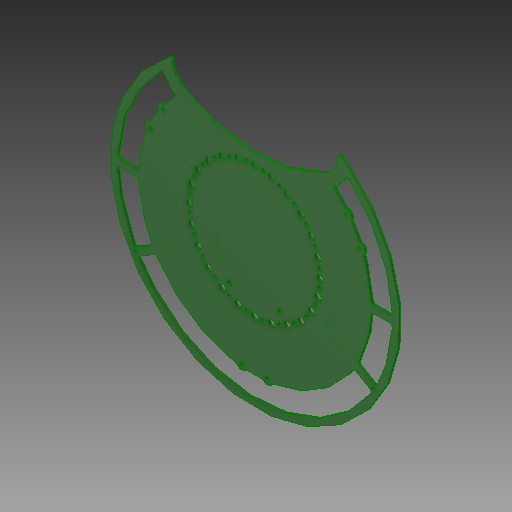
# Autodesk Inventor part: Board 0.brd_Outline
Saved by Autodesk Inventor 2017 (Build 210142000, 142)
## iProperties
Created: 2019-06-13
Part Number: Board 0.brd_Outline
Material: Generic
Document SubType Name: Modeling
Designer: Marc
Density: 1 g/cm^3
Appearance: Board Outline
Author: Marc
Autodesk Inventor part; units mm, degrees
ref_plane "YZ Plane" through (0, 0, 0) normal (1, 0, 0) x (0, 1, 0)
ref_plane "XZ Plane" through (0, 0, 0) normal (0, 1, 0) x (-1, 0, 0)
ref_plane "XY Plane" through (0, 0, 0) normal (0, 0, 1) x (1, 0, 0)
sketch "Sketch1" plane through (0, 0, 0) normal (0, 0, 1) x (1, 0, 0)
  line L0 (-60.7484, 83.79) -> (-60.8086, 84.044)
  line L1 (-60.8086, 84.044) -> (-60.9324, 84.2738)
  line L2 (-60.9324, 84.2738) -> (-61.1115, 84.4637)
  line L3 (-61.1115, 84.4637) -> (-61.3337, 84.6008)
  line L4 (-61.3337, 84.6008) -> (-61.5837, 84.6757)
  line L5 (-61.5837, 84.6757) -> (-61.8447, 84.6834)
  line L6 (-61.8447, 84.6834) -> (-62.0987, 84.6232)
  line L7 (-62.0987, 84.6232) -> (-62.3285, 84.4994)
  line L8 (-62.3285, 84.4994) -> (-62.337, 84.4932)
  line L9 (-62.337, 84.4932) -> (-82.0805, 65.4803)
  line L10 (-82.0805, 65.4803) -> (-96.2304, 42.0052)
  line L11 (-96.2304, 42.0052) -> (-103.8223, 15.6678)
  line L12 (-103.8223, 15.6678) -> (-104.339, -11.7372)
  line L13 (-104.339, -11.7372) -> (-97.7451, -38.342)
  line L14 (-97.7451, -38.342) -> (-84.49, -62.3337)
  line L15 (-84.49, -62.3337) -> (-65.4771, -82.0773)
  line L16 (-65.4771, -82.0773) -> (-42.002, -96.2272)
  line L17 (-42.002, -96.2272) -> (-15.6646, -103.8191)
  line L18 (-15.6646, -103.8191) -> (11.7404, -104.3358)
  line L19 (11.7404, -104.3358) -> (38.3452, -97.7419)
  line L20 (38.3452, -97.7419) -> (62.3369, -84.4868)
  line L21 (62.3369, -84.4868) -> (82.0805, -65.4739)
  line L22 (82.0805, -65.4739) -> (96.2304, -41.9988)
  line L23 (96.2304, -41.9988) -> (103.8223, -15.6614)
  line L24 (103.8223, -15.6614) -> (104.339, 11.7436)
  line L25 (104.339, 11.7436) -> (97.7451, 38.3484)
  line L26 (97.7451, 38.3484) -> (84.49, 62.3401)
  line L27 (84.49, 62.3401) -> (65.4771, 82.0837)
  line L28 (65.4771, 82.0837) -> (62.337, 84.4932)
  line L29 (62.337, 84.4932) -> (62.1085, 84.6195)
  line L30 (62.1085, 84.6195) -> (61.8551, 84.6823)
  line L31 (61.8551, 84.6823) -> (61.5941, 84.6773)
  line L32 (61.5941, 84.6773) -> (61.3432, 84.605)
  line L33 (61.3432, 84.605) -> (61.1197, 84.4703)
  line L34 (61.1197, 84.4703) -> (60.9386, 84.2823)
  line L35 (60.9386, 84.2823) -> (60.8123, 84.0538)
  line L36 (60.8123, 84.0538) -> (60.7495, 83.8004)
  line L37 (60.7495, 83.8004) -> (60.7484, 83.79)
  line L38 (60.7484, 83.79) -> (59.5017, 78.5255)
  line L39 (59.5017, 78.5255) -> (56.935, 73.7631)
  line L40 (56.935, 73.7631) -> (53.2231, 69.8273)
  line L41 (53.2231, 69.8273) -> (50, 67.6691)
  line L42 (50, 67.6691) -> (24.3974, 57.8745)
  line L43 (24.3974, 57.8745) -> (-2.8678, 55.04)
  line L44 (-2.8678, 55.04) -> (-29.9376, 59.359)
  line L45 (-29.9376, 59.359) -> (-50, 67.6691)
  line L46 (-50, 67.6691) -> (-54.3803, 70.8442)
  line L47 (-54.3803, 70.8442) -> (-57.7896, 75.0449)
  line L48 (-57.7896, 75.0449) -> (-59.9955, 79.9848)
  line L49 (-59.9955, 79.9848) -> (-60.7484, 83.79)
  line L50 (-83.531, -51.1134) -> (-73.5598, -45.3565)
  line L51 (-73.5598, -45.3565) -> (-73.0774, -45.1567)
  line L52 (-73.0774, -45.1567) -> (-72.5598, -45.0885)
  line L53 (-72.5598, -45.0885) -> (-72.0422, -45.1567)
  line L54 (-72.0422, -45.1567) -> (-71.5598, -45.3565)
  line L55 (-71.5598, -45.3565) -> (-71.1456, -45.6743)
  line L56 (-71.1456, -45.6743) -> (-70.8821, -45.9998)
  line L57 (-70.8821, -45.9998) -> (-56.5631, -62.7771)
  line L58 (-56.5631, -62.7771) -> (-38.3898, -75.2767)
  line L59 (-38.3898, -75.2767) -> (-17.6006, -82.6468)
  line L60 (-17.6006, -82.6468) -> (-13.0912, -83.4798)
  line L61 (-13.0912, -83.4798) -> (-12.5816, -84.3912)
  line L62 (-12.5816, -84.3912) -> (-11.8534, -85.1396)
  line L63 (-11.8534, -85.1396) -> (-10.9564, -85.6741)
  line L64 (-10.9564, -85.6741) -> (-9.9515, -85.9582)
  line L65 (-9.9515, -85.9582) -> (-8.9074, -85.9725)
  line L66 (-8.9074, -85.9725) -> (-7.8952, -85.7162)
  line L67 (-7.8952, -85.7162) -> (-6.9838, -85.2065)
  line L68 (-6.9838, -85.2065) -> (-6.2353, -84.4784)
  line L69 (-6.2353, -84.4784) -> (-6.0887, -84.2803)
  line L70 (-6.0887, -84.2803) -> (6.0887, -84.2803)
  line L71 (6.0887, -84.2803) -> (6.7909, -85.0532)
  line L72 (6.7909, -85.0532) -> (7.6692, -85.618)
  line L73 (7.6692, -85.618) -> (8.6637, -85.9362)
  line L74 (8.6637, -85.9362) -> (9.7067, -85.9862)
  line L75 (9.7067, -85.9862) -> (10.7271, -85.7645)
  line L76 (10.7271, -85.7645) -> (11.6554, -85.2863)
  line L77 (11.6554, -85.2863) -> (12.4283, -84.5841)
  line L78 (12.4283, -84.5841) -> (12.9931, -83.7058)
  line L79 (12.9931, -83.7058) -> (13.0912, -83.4798)
  line L80 (13.0912, -83.4798) -> (34.2497, -77.2484)
  line L81 (34.2497, -77.2484) -> (53.0744, -65.7531)
  line L82 (53.0744, -65.7531) -> (68.2824, -49.7774)
  line L83 (68.2824, -49.7774) -> (70.8821, -45.9998)
  line L84 (70.8821, -45.9998) -> (71.221, -45.6027)
  line L85 (71.221, -45.6027) -> (71.6512, -45.3068)
  line L86 (71.6512, -45.3068) -> (72.1433, -45.1324)
  line L87 (72.1433, -45.1324) -> (72.6638, -45.0912)
  line L88 (72.6638, -45.0912) -> (73.1771, -45.1862)
  line L89 (73.1771, -45.1862) -> (73.5598, -45.3565)
  line L90 (73.5598, -45.3565) -> (83.531, -51.1134)
  line L91 (83.531, -51.1134) -> (83.9452, -51.4312)
  line L92 (83.9452, -51.4312) -> (84.263, -51.8455)
  line L93 (84.263, -51.8455) -> (84.4628, -52.3278)
  line L94 (84.4628, -52.3278) -> (84.531, -52.8455)
  line L95 (84.531, -52.8455) -> (84.4628, -53.3631)
  line L96 (84.4628, -53.3631) -> (84.263, -53.8455)
  line L97 (84.263, -53.8455) -> (84.2153, -53.9239)
  line L98 (84.2153, -53.9239) -> (67.3902, -73.8831)
  line L99 (67.3902, -73.8831) -> (45.9725, -88.8076)
  line L100 (45.9725, -88.8076) -> (21.4219, -97.6803)
  line L101 (21.4219, -97.6803) -> (-4.5885, -99.8964)
  line L102 (-4.5885, -99.8964) -> (-30.2863, -95.3051)
  line L103 (-30.2863, -95.3051) -> (-53.9201, -84.2191)
  line L104 (-53.9201, -84.2191) -> (-73.8793, -67.394)
  line L105 (-73.8793, -67.394) -> (-84.2153, -53.9239)
  line L106 (-84.2153, -53.9239) -> (-84.437, -53.4512)
  line L107 (-84.437, -53.4512) -> (-84.5288, -52.9373)
  line L108 (-84.5288, -52.9373) -> (-84.4845, -52.417)
  line L109 (-84.4845, -52.417) -> (-84.3071, -51.926)
  line L110 (-84.3071, -51.926) -> (-84.0086, -51.4976)
  line L111 (-84.0086, -51.4976) -> (-83.6094, -51.1611)
  line L112 (-83.6094, -51.1611) -> (-83.531, -51.1134)
  line L113 (-76.0333, 36.8672) -> (-77.0537, 36.6456)
  line L114 (-77.0537, 36.6456) -> (-77.9819, 36.1673)
  line L115 (-77.9819, 36.1673) -> (-78.7548, 35.4651)
  line L116 (-78.7548, 35.4651) -> (-79.3196, 34.5868)
  line L117 (-79.3196, 34.5868) -> (-79.6378, 33.5923)
  line L118 (-79.6378, 33.5923) -> (-79.6878, 32.5492)
  line L119 (-79.6878, 32.5492) -> (-79.4661, 31.5288)
  line L120 (-79.4661, 31.5288) -> (-78.9878, 30.6006)
  line L121 (-78.9878, 30.6006) -> (-78.8412, 30.4026)
  line L122 (-78.8412, 30.4026) -> (-84.0231, 8.9665)
  line L123 (-84.0231, 8.9665) -> (-84.3856, 4.396)
  line L124 (-84.3856, 4.396) -> (-84.4806, 3.8826)
  line L125 (-84.4806, 3.8826) -> (-84.7052, 3.4113)
  line L126 (-84.7052, 3.4113) -> (-85.0441, 3.0141)
  line L127 (-85.0441, 3.0141) -> (-85.4743, 2.7183)
  line L128 (-85.4743, 2.7183) -> (-85.9664, 2.5438)
  line L129 (-85.9664, 2.5438) -> (-86.3829, 2.5)
  line L130 (-86.3829, 2.5) -> (-97.8966, 2.5)
  line L131 (-97.8966, 2.5) -> (-98.4143, 2.5682)
  line L132 (-98.4143, 2.5682) -> (-98.8966, 2.768)
  line L133 (-98.8966, 2.768) -> (-99.3109, 3.0858)
  line L134 (-99.3109, 3.0858) -> (-99.6287, 3.5)
  line L135 (-99.6287, 3.5) -> (-99.8285, 3.9824)
  line L136 (-99.8285, 3.9824) -> (-99.8966, 4.5001)
  line L137 (-99.8966, 4.5001) -> (-99.8945, 4.5918)
  line L138 (-99.8945, 4.5918) -> (-95.3026, 30.2894)
  line L139 (-95.3026, 30.2894) -> (-84.2162, 53.9228)
  line L140 (-84.2162, 53.9228) -> (-68.6444, 72.7182)
  line L141 (-68.6444, 72.7182) -> (-68.2212, 73.024)
  line L142 (-68.2212, 73.024) -> (-67.7333, 73.2098)
  line L143 (-67.7333, 73.2098) -> (-67.2139, 73.263)
  line L144 (-67.2139, 73.263) -> (-66.6984, 73.1799)
  line L145 (-66.6984, 73.1799) -> (-66.222, 72.9663)
  line L146 (-66.222, 72.9663) -> (-65.8171, 72.6366)
  line L147 (-65.8171, 72.6366) -> (-65.5113, 72.2134)
  line L148 (-65.5113, 72.2134) -> (-65.511, 72.2128)
  line L149 (-65.511, 72.2128) -> (-61.1063, 66.1109)
  line L150 (-61.1063, 66.1109) -> (-59.4525, 64.4927)
  line L151 (-59.4525, 64.4927) -> (-58.8449, 64.1171)
  line L152 (-58.8449, 64.1171) -> (-58.4393, 63.7882)
  line L153 (-58.4393, 63.7882) -> (-58.1327, 63.3656)
  line L154 (-58.1327, 63.3656) -> (-57.9459, 62.8781)
  line L155 (-57.9459, 62.8781) -> (-57.8917, 62.3588)
  line L156 (-57.8917, 62.3588) -> (-57.9738, 61.8431)
  line L157 (-57.9738, 61.8431) -> (-58.1865, 61.3663)
  line L158 (-58.1865, 61.3663) -> (-58.5062, 60.9694)
  line L159 (-58.5062, 60.9694) -> (-65.75, 53.0772)
  line L160 (-65.75, 53.0772) -> (-66.7941, 53.0916)
  line L161 (-66.7941, 53.0916) -> (-67.8064, 52.8352)
  line L162 (-67.8064, 52.8352) -> (-68.7178, 52.3255)
  line L163 (-68.7178, 52.3255) -> (-69.4662, 51.5974)
  line L164 (-69.4662, 51.5974) -> (-70.0007, 50.7003)
  line L165 (-70.0007, 50.7003) -> (-70.2848, 49.6955)
  line L166 (-70.2848, 49.6955) -> (-70.2991, 48.6514)
  line L167 (-70.2991, 48.6514) -> (-70.0428, 47.6391)
  line L168 (-70.0428, 47.6391) -> (-69.9446, 47.4131)
  line L169 (-69.9446, 47.4131) -> (-76.0333, 36.8672)
  line L170 (97.8966, 2.5) -> (86.3829, 2.5)
  line L171 (86.3829, 2.5) -> (85.8652, 2.5681)
  line L172 (85.8652, 2.5681) -> (85.3829, 2.7679)
  line L173 (85.3829, 2.7679) -> (84.9687, 3.0857)
  line L174 (84.9687, 3.0857) -> (84.6508, 3.4999)
  line L175 (84.6508, 3.4999) -> (84.451, 3.9823)
  line L176 (84.451, 3.9823) -> (84.3856, 4.396)
  line L177 (84.3856, 4.396) -> (80.3743, 26.0815)
  line L178 (80.3743, 26.0815) -> (78.8412, 30.4026)
  line L179 (78.8412, 30.4026) -> (79.3757, 31.2996)
  line L180 (79.3757, 31.2996) -> (79.6598, 32.3044)
  line L181 (79.6598, 32.3044) -> (79.6741, 33.3486)
  line L182 (79.6741, 33.3486) -> (79.4177, 34.3608)
  line L183 (79.4177, 34.3608) -> (78.9081, 35.2722)
  line L184 (78.9081, 35.2722) -> (78.18, 36.0207)
  line L185 (78.18, 36.0207) -> (77.2829, 36.5552)
  line L186 (77.2829, 36.5552) -> (76.2781, 36.8393)
  line L187 (76.2781, 36.8393) -> (76.0333, 36.8672)
  line L188 (76.0333, 36.8672) -> (69.9446, 47.4131)
  line L189 (69.9446, 47.4131) -> (70.2628, 48.4077)
  line L190 (70.2628, 48.4077) -> (70.3128, 49.4507)
  line L191 (70.3128, 49.4507) -> (70.0911, 50.4711)
  line L192 (70.0911, 50.4711) -> (69.6129, 51.3994)
  line L193 (69.6129, 51.3994) -> (68.9107, 52.1722)
  line L194 (68.9107, 52.1722) -> (68.0324, 52.737)
  line L195 (68.0324, 52.737) -> (67.0378, 53.0552)
  line L196 (67.0378, 53.0552) -> (65.9948, 53.1052)
  line L197 (65.9948, 53.1052) -> (65.75, 53.0772)
  line L198 (65.75, 53.0772) -> (58.5062, 60.9694)
  line L199 (58.5062, 60.9694) -> (58.1799, 61.377)
  line L200 (58.1799, 61.377) -> (57.9702, 61.8552)
  line L201 (57.9702, 61.8552) -> (57.8914, 62.3713)
  line L202 (57.8914, 62.3713) -> (57.9489, 62.8903)
  line L203 (57.9489, 62.8903) -> (58.1387, 63.3766)
  line L204 (58.1387, 63.3766) -> (58.448, 63.7973)
  line L205 (58.448, 63.7973) -> (58.8449, 64.1171)
  line L206 (58.8449, 64.1171) -> (59.4525, 64.4927)
  line L207 (59.4525, 64.4927) -> (64.3323, 70.2217)
  line L208 (64.3323, 70.2217) -> (65.511, 72.2128)
  line L209 (65.511, 72.2128) -> (65.8166, 72.6361)
  line L210 (65.8166, 72.6361) -> (66.2214, 72.9659)
  line L211 (66.2214, 72.9659) -> (66.6977, 73.1797)
  line L212 (66.6977, 73.1797) -> (67.2132, 73.263)
  line L213 (67.2132, 73.263) -> (67.7326, 73.21)
  line L214 (67.7326, 73.21) -> (68.2206, 73.0243)
  line L215 (68.2206, 73.0243) -> (68.6439, 72.7187)
  line L216 (68.6439, 72.7187) -> (68.6444, 72.7182)
  line L217 (68.6444, 72.7182) -> (85.1261, 52.4746)
  line L218 (85.1261, 52.4746) -> (95.8067, 28.655)
  line L219 (95.8067, 28.655) -> (99.8945, 4.5918)
  line L220 (99.8945, 4.5918) -> (99.8502, 4.0716)
  line L221 (99.8502, 4.0716) -> (99.6728, 3.5806)
  line L222 (99.6728, 3.5806) -> (99.3743, 3.1522)
  line L223 (99.3743, 3.1522) -> (98.9751, 2.8157)
  line L224 (98.9751, 2.8157) -> (98.5024, 2.5939)
  line L225 (98.5024, 2.5939) -> (97.9884, 2.5021)
  line L226 (97.9884, 2.5021) -> (97.8966, 2.5)
  line L227 (-97.8966, -2.5) -> (-86.3829, -2.5)
  line L228 (-86.3829, -2.5) -> (-85.8652, -2.5681)
  line L229 (-85.8652, -2.5681) -> (-85.3829, -2.7679)
  line L230 (-85.3829, -2.7679) -> (-84.9687, -3.0857)
  line L231 (-84.9687, -3.0857) -> (-84.6508, -3.4999)
  line L232 (-84.6508, -3.4999) -> (-84.451, -3.9823)
  line L233 (-84.451, -3.9823) -> (-84.3856, -4.396)
  line L234 (-84.3856, -4.396) -> (-80.3739, -26.0833)
  line L235 (-80.3739, -26.0833) -> (-75.278, -38.3858)
  line L236 (-75.278, -38.3858) -> (-75.1036, -38.8779)
  line L237 (-75.1036, -38.8779) -> (-75.0625, -39.3983)
  line L238 (-75.0625, -39.3983) -> (-75.1574, -39.9117)
  line L239 (-75.1574, -39.9117) -> (-75.382, -40.383)
  line L240 (-75.382, -40.383) -> (-75.721, -40.7802)
  line L241 (-75.721, -40.7802) -> (-76.0598, -41.0264)
  line L242 (-76.0598, -41.0264) -> (-86.031, -46.7833)
  line L243 (-86.031, -46.7833) -> (-86.5133, -46.983)
  line L244 (-86.5133, -46.983) -> (-87.031, -47.0512)
  line L245 (-87.031, -47.0512) -> (-87.5486, -46.983)
  line L246 (-87.5486, -46.983) -> (-88.031, -46.7832)
  line L247 (-88.031, -46.7832) -> (-88.4452, -46.4654)
  line L248 (-88.4452, -46.4654) -> (-88.763, -46.0511)
  line L249 (-88.763, -46.0511) -> (-88.8071, -45.9706)
  line L250 (-88.8071, -45.9706) -> (-97.6786, -21.4231)
  line L251 (-97.6786, -21.4231) -> (-99.8945, -4.5918)
  line L252 (-99.8945, -4.5918) -> (-99.8502, -4.0716)
  line L253 (-99.8502, -4.0716) -> (-99.6728, -3.5806)
  line L254 (-99.6728, -3.5806) -> (-99.3743, -3.1522)
  line L255 (-99.3743, -3.1522) -> (-98.9751, -2.8157)
  line L256 (-98.9751, -2.8157) -> (-98.5024, -2.5939)
  line L257 (-98.5024, -2.5939) -> (-97.9884, -2.5021)
  line L258 (-97.9884, -2.5021) -> (-97.8966, -2.5)
  line L259 (86.031, -46.7833) -> (76.0598, -41.0264)
  line L260 (76.0598, -41.0264) -> (75.6456, -40.7085)
  line L261 (75.6456, -40.7085) -> (75.3277, -40.2943)
  line L262 (75.3277, -40.2943) -> (75.1279, -39.812)
  line L263 (75.1279, -39.812) -> (75.0597, -39.2944)
  line L264 (75.0597, -39.2944) -> (75.1279, -38.7767)
  line L265 (75.1279, -38.7767) -> (75.278, -38.3858)
  line L266 (75.278, -38.3858) -> (82.6475, -17.5982)
  line L267 (82.6475, -17.5982) -> (84.3856, -4.396)
  line L268 (84.3856, -4.396) -> (84.4806, -3.8826)
  line L269 (84.4806, -3.8826) -> (84.7052, -3.4113)
  line L270 (84.7052, -3.4113) -> (85.0441, -3.0141)
  line L271 (85.0441, -3.0141) -> (85.4743, -2.7183)
  line L272 (85.4743, -2.7183) -> (85.9664, -2.5438)
  line L273 (85.9664, -2.5438) -> (86.3829, -2.5)
  line L274 (86.3829, -2.5) -> (97.8966, -2.5)
  line L275 (97.8966, -2.5) -> (98.4143, -2.5682)
  line L276 (98.4143, -2.5682) -> (98.8966, -2.768)
  line L277 (98.8966, -2.768) -> (99.3109, -3.0858)
  line L278 (99.3109, -3.0858) -> (99.6287, -3.5)
  line L279 (99.6287, -3.5) -> (99.8285, -3.9824)
  line L280 (99.8285, -3.9824) -> (99.8966, -4.5001)
  line L281 (99.8966, -4.5001) -> (99.8945, -4.5918)
  line L282 (99.8945, -4.5918) -> (95.3037, -30.2863)
  line L283 (95.3037, -30.2863) -> (88.8071, -45.9706)
  line L284 (88.8071, -45.9706) -> (88.5086, -46.399)
  line L285 (88.5086, -46.399) -> (88.1094, -46.7355)
  line L286 (88.1094, -46.7355) -> (87.6367, -46.9572)
  line L287 (87.6367, -46.9572) -> (87.1228, -47.0491)
  line L288 (87.1228, -47.0491) -> (86.6025, -47.0048)
  line L289 (86.6025, -47.0048) -> (86.1115, -46.8273)
  line L290 (86.1115, -46.8273) -> (86.031, -46.7833)
  circle A0 centre (-75.7016, 32.881) radius 1.5
  circle A1 centre (-66.3266, 49.119) radius 1.5
  circle A2 centre (66.3266, 49.119) radius 1.5
  circle A3 centre (75.7016, 32.881) radius 1.5
  circle A4 centre (86.5112, -49.9473) radius 1.5
  circle A5 centre (-86.5112, -49.9473) radius 1.5
  circle A6 centre (-9.375, -82) radius 1.5
  circle A7 centre (9.375, -82) radius 1.5
  circle A8 centre (-18.1775, -35.3843) radius 1.5
  circle A9 centre (18.1775, -35.3843) radius 1.5
  circle A10 centre (-47.0936, 6.2) radius 1.55
  circle A11 centre (-43.8843, 18.1775) radius 1.55
  circle A12 centre (-37.6843, 28.9162) radius 1.55
  circle A13 centre (-28.9162, 37.6843) radius 1.55
  circle A14 centre (-18.1775, 43.8843) radius 1.55
  circle A15 centre (-6.2, 47.0936) radius 1.55
  circle A16 centre (-6.2, -47.0936) radius 1.55
  circle A17 centre (-18.1775, -43.8843) radius 1.55
  circle A18 centre (-28.9162, -37.6843) radius 1.55
  circle A19 centre (-37.6843, -28.9162) radius 1.55
  circle A20 centre (-43.8843, -18.1775) radius 1.55
  circle A21 centre (-47.0936, -6.2) radius 1.55
  circle A22 centre (47.0936, -6.2) radius 1.55
  circle A23 centre (43.8843, -18.1775) radius 1.55
  circle A24 centre (37.6843, -28.9162) radius 1.55
  circle A25 centre (28.9162, -37.6843) radius 1.55
  circle A26 centre (18.1775, -43.8843) radius 1.55
  circle A27 centre (6.2, -47.0936) radius 1.55
  circle A28 centre (6.2, 47.0936) radius 1.55
  circle A29 centre (18.1775, 43.8843) radius 1.55
  circle A30 centre (28.9162, 37.6843) radius 1.55
  circle A31 centre (37.6843, 28.9162) radius 1.55
  circle A32 centre (43.8843, 18.1775) radius 1.55
  circle A33 centre (47.0936, 6.2) radius 1.55
  circle A34 centre (-47.5, 0) radius 2.5
  circle A35 centre (-45.8815, 12.2939) radius 2.5
  circle A36 centre (-41.1362, 23.75) radius 2.5
  circle A37 centre (-33.5876, 33.5876) radius 2.5
  circle A38 centre (-23.75, 41.1362) radius 2.5
  circle A39 centre (-12.2939, 45.8815) radius 2.5
  circle A40 centre (0, -47.5) radius 2.5
  circle A41 centre (-12.2939, -45.8815) radius 2.5
  circle A42 centre (-23.75, -41.1362) radius 2.5
  circle A43 centre (-33.5876, -33.5876) radius 2.5
  circle A44 centre (-41.1362, -23.75) radius 2.5
  circle A45 centre (-45.8815, -12.2939) radius 2.5
  circle A46 centre (47.5, 0) radius 2.5
  circle A47 centre (45.8815, -12.2939) radius 2.5
  circle A48 centre (41.1362, -23.75) radius 2.5
  circle A49 centre (33.5876, -33.5876) radius 2.5
  circle A50 centre (23.75, -41.1362) radius 2.5
  circle A51 centre (12.2939, -45.8815) radius 2.5
  circle A52 centre (0, 47.5) radius 2.5
  circle A53 centre (12.2939, 45.8815) radius 2.5
  circle A54 centre (23.75, 41.1362) radius 2.5
  circle A55 centre (33.5876, 33.5876) radius 2.5
  circle A56 centre (41.1362, 23.75) radius 2.5
  circle A57 centre (45.8815, 12.2939) radius 2.5
  circle A58 centre (-38.1762, -33.7185) radius 0.3048
  circle A59 centre (-36.6903, -42.4053) radius 0.3048
  circle A60 centre (-24.2316, -48.4632) radius 0.3048
  circle A61 centre (-31.4325, -51.2064) radius 0.3048
  circle A62 centre (-72.1233, -21.9456) radius 0.3048
  circle A63 centre (-73.9521, -20.1168) radius 0.3048
  circle A64 centre (-56.4642, -5.715) radius 0.3048
  circle A65 centre (-60.2361, -5.715) radius 0.3048
  circle A66 centre (-54.6354, 6.6294) radius 0.3048
  circle A67 centre (-51.435, -17.145) radius 0.3048
  circle A68 centre (-57.9501, 13.8303) radius 0.3048
  circle A69 centre (52.2351, -27.8892) radius 0.3048
  circle A70 centre (52.2351, -25.8318) radius 0.3048
  circle A71 centre (48.9204, -33.6042) radius 0.3048
  circle A72 centre (-23.2029, -24.2316) radius 0.3048
  circle A73 centre (-26.5176, -19.431) radius 0.3048
  circle A74 centre (58.5216, -33.6042) radius 0.175
  circle A75 centre (1.2573, -56.2356) radius 0.175
  circle A76 centre (57.15, -32.1183) radius 0.175
  circle A77 centre (16.002, -54.1782) radius 0.175
  circle A78 centre (54.0639, -29.6037) radius 0.175
  circle A79 centre (39.8907, -41.9481) radius 0.175
  circle A80 centre (49.3776, -32.3469) radius 0.175
  circle A81 centre (49.3776, -16.5735) radius 0.175
  circle A82 centre (62.5221, -28.1178) radius 0.175
  circle A83 centre (58.293, -1.4859) radius 0.175
  circle A84 centre (57.0357, -26.1747) radius 0.175
  circle A85 centre (51.435, 10.8585) radius 0.175
  circle A86 centre (54.2925, 13.6017) radius 0.175
  circle A87 centre (-26.289, -17.0307) radius 0.175
  circle A88 centre (31.4325, 17.7165) radius 0.175
  circle A89 centre (-24.6888, -11.7729) radius 0.175
  circle A90 centre (25.4889, 25.4889) radius 0.175
  circle A91 centre (29.1465, 27.6606) radius 0.175
  circle A92 centre (-26.4033, -12.573) radius 0.175
  circle A93 centre (17.9451, 31.2039) radius 0.175
  circle A94 centre (20.8026, 35.6616) radius 0.175
  circle A95 centre (-27.0891, -11.8872) radius 0.175
  circle A96 centre (8.4582, 34.9758) radius 0.175
  circle A97 centre (10.9728, 40.1193) radius 0.175
  circle A98 centre (-27.8892, -12.4587) radius 0.175
  circle A99 centre (-1.4859, 37.3761) radius 0.175
  circle A100 centre (1.0287, 40.1193) radius 0.175
  circle A101 centre (-28.6893, -11.7729) radius 0.175
  circle A102 centre (-9.4869, 34.7472) radius 0.175
  circle A103 centre (-8.9154, 39.0906) radius 0.175
  circle A104 centre (-28.6893, -20.3454) radius 0.175
  circle A105 centre (-19.7739, 31.3182) radius 0.175
  circle A106 centre (-26.9748, -16.2306) radius 0.175
  circle A107 centre (-25.7175, -11.8872) radius 0.175
  circle A108 centre (-26.1747, -8.2296) radius 0.175
  circle A109 centre (-26.1747, 22.9743) radius 0.175
  circle A110 centre (-59.436, -33.3756) radius 0.175
  circle A111 centre (-49.8348, 27.0891) radius 0.175
  circle A112 centre (-58.6359, -41.7195) radius 0.175
  circle A113 centre (-70.9803, -8.9154) radius 0.175
  circle A114 centre (-49.6062, -37.6047) radius 0.175
  circle A115 centre (-54.4068, -16.1163) radius 0.175
  circle A116 centre (-58.5216, -37.6047) radius 0.175
  circle A117 centre (-42.291, -41.0337) radius 0.175
  circle A118 centre (-45.1485, -41.0337) radius 0.175
  circle A119 centre (-32.4612, -49.6062) radius 0.175
  circle A120 centre (-30.1752, -49.3776) radius 0.175
  circle A121 centre (-25.3746, -23.3172) radius 0.175
  circle A122 centre (21.4884, -7.6581) radius 0.175
  circle A123 centre (-65.4939, -39.8907) radius 0.175
  circle A124 centre (-39.4335, -65.9511) radius 0.175
  circle A125 centre (66.8655, -37.8333) radius 0.175
  circle A126 centre (32.6898, -67.6656) radius 0.175
  circle A127 centre (-27.0891, -25.7175) radius 0.175
  circle A128 centre (35.7759, -11.2014) radius 0.175
  circle A129 centre (17.3736, -12.8016) radius 0.175
  circle A130 centre (-30.9753, -16.9164) radius 0.175
  circle A131 centre (-54.4068, -35.7759) radius 0.175
  circle A132 centre (-46.5201, -31.8897) radius 0.175
  circle A133 centre (-44.1198, -34.29) radius 0.175
  circle A134 centre (-37.6047, -55.3212) radius 0.175
  circle A135 centre (67.5513, -33.6042) radius 0.175
  circle A136 centre (53.3781, -55.6641) radius 0.175
  circle A137 centre (-22.6314, -21.9456) radius 0.175
  circle A138 centre (6.1722, -21.9456) radius 0.175
  circle A139 centre (17.8308, -10.1727) radius 0.175
  circle A140 centre (-62.6364, -27.3177) radius 0.175
  circle A141 centre (-69.6087, -4.9149) radius 0.175
  circle A142 centre (64.2366, -33.3756) radius 0.175
  circle A143 centre (72.5805, 10.4013) radius 0.175
  circle A144 centre (-60.1218, -34.0614) radius 0.175
  circle A145 centre (-71.3232, -2.4003) radius 0.175
  circle A146 centre (60.1218, -38.5191) radius 0.175
  circle A147 centre (72.2376, 7.7724) radius 0.175
  circle A148 centre (-36.1188, -15.7734) radius 0.175
  circle A149 centre (-39.5478, -3.6576) radius 0.175
  circle A150 centre (-64.8081, -4.0005) radius 0.3048
  circle A151 centre (-68.58, -0.2286) radius 0.3048
  circle A152 centre (60.8076, -35.5473) radius 0.3048
  circle A153 centre (62.865, -33.4899) radius 0.3048
  circle A154 centre (55.8927, -26.4033) radius 0.3048
  circle A155 centre (55.7784, -17.9451) radius 0.3048
  circle A156 centre (4.2291, -59.7789) radius 0.3048
  circle A157 centre (2.4003, -57.9501) radius 0.3048
  circle A158 centre (49.2633, -35.6616) radius 0.3048
  circle A159 centre (-26.5176, -21.2598) radius 0.3048
  circle A160 centre (-29.3751, -18.4023) radius 0.3048
  circle A161 centre (-21.4884, -13.4874) radius 0.3048
  circle A162 centre (-50.7492, 25.146) radius 0.3048
  circle A163 centre (-52.8066, 24.5745) radius 0.3048
  circle A164 centre (-62.1792, -38.1762) radius 0.3048
  circle A165 centre (-60.8076, -36.8046) radius 0.3048
  circle A166 centre (-53.0352, -36.6903) radius 0.3048
  circle A167 centre (-45.2628, -31.5468) radius 0.3048
  circle A168 centre (-60.9219, -14.7447) radius 0.3048
  circle A169 centre (-39.7764, -39.4335) radius 0.3048
  circle A170 centre (-52.6923, 14.0589) radius 0.3048
  constraints: 582 end point, 171 centre point
extrude "Board 0.brd_Outline" add sketch "Sketch1" along normal blind 1.6
body "Solid1"
